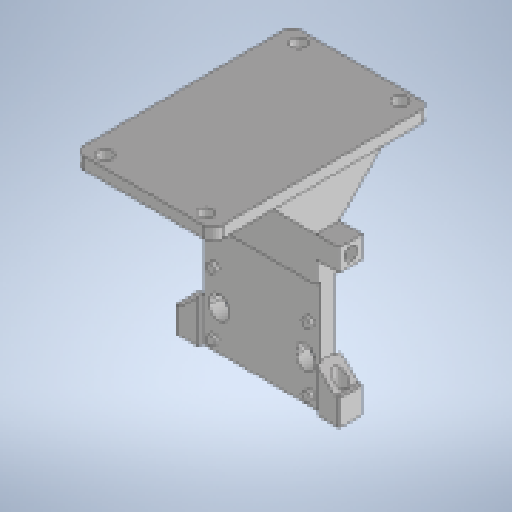
# Autodesk Inventor part: cameraholder
Saved by Autodesk Inventor 2025.1 (Build 291241000, 241)
## iProperties
Created: 2026-04-04
Part Number: cameraholder
Material: Generic
Document SubType Name: Modeling
Designer: User
Density: 1 g/cm^3
Appearance: Default
Author: User
## iProperties of the stored document cameraholder_3DPrint.ipt
Created: 2026-04-04
Part Number: cameraholder_3DPrint
Material: Generic
Document SubType Name: Modeling
Designer: User
Density: 1 g/cm^3
Appearance: Default
Author: User
Autodesk Inventor part; units mm, degrees
ref_plane "YZ Plane" through (0, 0, 0) normal (1, 0, 0) x (0, 1, 0)
sketch "Sketch1" plane through (0, 0, 0) normal (0, 0, 1) x (1, 0, 0)
  circle A0 centre (10.25, -9.75) radius 1.1 projected
  circle A1 centre (-10.25, -9.75) radius 1.1 projected
  circle A2 centre (-10.25, 3.75) radius 1.1 projected
  circle A3 centre (10.25, 3.75) radius 1.1 projected
  circle A4 centre (9.25, -4) radius 1.5 projected
  circle A5 centre (-9.25, -4) radius 1.5 projected
  arc A6 (7.25, -4) -> (11.25, -4) centre (9.25, -4) ccw
  arc A7 (-11.25, -4) -> (-7.25, -4) centre (-9.25, -4) ccw
  line L0 (8.2, -12) -> (-8.2, -12) projected
  line L1 (12.5, 1) -> (12.5, -7.7) projected
  line L2 (-12.5, 12) -> (12.5, 12) projected
  line L3 (-12.5, -7.7) -> (-12.5, 1) projected
  line L4 (12.5, -12) -> (-12.5, -12)
  line L5 (-12.5, -12) -> (-12.5, 12)
  line L6 (-12.5, 12) -> (12.5, 12)
  line L7 (12.5, 12) -> (12.5, -12)
  line L8 (-9.25, -4) -> (-9.25, -3)
  line L9 (9.25, -4) -> (9.25, -3)
  line L10 (-11.25, -4) -> (-11.25, -3)
  line L11 (-7.25, -4) -> (-7.25, -3)
  line L12 (7.25, -4) -> (7.25, -3)
  line L13 (11.25, -4) -> (11.25, -3)
  arc A8 (-9.25, -5) -> (-7.7976, -4.375) centre (-9.25, -3) ccw
  arc A9 (-7.25, -3) -> (-11.25, -3) centre (-9.25, -3) ccw
  arc A10 (9.25, -5) -> (10.7024, -4.375) centre (9.25, -3) ccw
  arc A11 (11.25, -3) -> (7.25, -3) centre (9.25, -3) ccw
  point P0 (0, 0)
  dimension "d0" = 0.5
  dimension "d1" = 0.5
  dimension "d70" = 1
  dimension "d74" = 3.25
  constraints: 20 end point, 12 point on circle, 6 centre point, 6 tangent, 4 vertical, 3 parallel, 2 point on line, 1 horizontal, 1 perpendicular, 4 other
  measures "d70" distance of L8.start L8.end
  measures "d74" distance from line of L1 L9.end
extrude "Extrusion1" add sketch "Sketch1" along normal blind 3 contours L0 L4 L5 L3 L2 L7 L1
sketch "Sketch2" plane through (-12.5, 12, 0) normal (0, 1, 0) x (1, 0, 0)
  line L0 (25, 0) -> (0, 0) projected
  line L1 (0, 0) -> (0, -3) projected
  line L2 (25, -3) -> (0, -3) projected
  line L3 (25, 0) -> (25, -3) projected
  point P0 (12.5, 0)
extrude "Extrusion2" add sketch "Sketch2" along normal blind 2
sketch "Sketch3" plane through (-12.5, 14, 0) normal (0, 1, 0) x (1, 0, 0)
  line L0 (0, 1) -> (25, 1) projected
  line L1 (25, 0) -> (0, 0) projected
  line L2 (0, -3) -> (25, -3) projected
  line L3 (0, -4) -> (25, -4)
  line L4 (0, 1) -> (25, 1)
  line L5 (25, 1) -> (25, -4)
  line L6 (25, -4) -> (0, -4)
  line L7 (0, -4) -> (0, 1)
  point P0 (12.5, 0)
  dimension "d6" = 1
  constraints: 10 end point, 3 parallel, 1 horizontal, 1 perpendicular
  measures "d6" distance between parallel lines of L2 L3
extrude "Extrusion3" add sketch "Sketch3" along normal blind 7.5
sketch "Sketch8" plane through (-12.5, -12, 0) normal (-1, 0, 0) x (0, 0, 1)
  line L0 (4, 24) -> (3, 24)
  line L1 (3, 26) -> (4, 26) projected
  line L2 (3, 0) -> (3, 26) projected
  line L3 (0, 0) -> (0, 26) projected
  line L4 (-1, 26) -> (0, 26) projected
  line L5 (4, 24.1) -> (3, 24.1)
  line L6 (4, 24.1) -> (-1, 24.1)
  line L7 (0, 24.1) -> (-1, 24.1)
  line L8 (-1, 24.1) -> (-1, 26)
  line L9 (-1, 26) -> (0, 26)
  line L10 (0, 26) -> (0, 24.1)
  line L11 (3, 24.1) -> (4, 24.1)
  line L12 (4, 24.1) -> (4, 26)
  line L13 (4, 26) -> (3, 26)
  line L14 (3, 26) -> (3, 24.1)
  point P0 (0, 12)
  dimension "d22" = 0.1
  constraints: 22 end point, 5 parallel, 4 horizontal, 2 perpendicular, 2 point on line, 2 other
  measures "d22" distance between parallel lines of L0 L5
extrude "Extrusion7" add sketch "Sketch8" against normal up to surface (25 mm away)
sketch "Sketch9" plane through (0, 0, 3) normal (0, 0, 1) x (1, 0, 0)
  circle A0 centre (10.25, -9.75) radius 1.1
  circle A1 centre (10.25, 3.75) radius 1.1
  circle A2 centre (-10.25, 3.75) radius 1.1
  circle A3 centre (-10.25, -9.75) radius 1.1
  circle A4 centre (-10.25, -9.75) radius 1
  circle A5 centre (-10.25, 3.75) radius 1
  circle A6 centre (10.25, 3.75) radius 1
  circle A7 centre (10.25, -9.75) radius 1
  point P0 (0, 0)
  dimension "d25" = 0.1
  dimension "d26" = 0.1
  dimension "d27" = 0.1
  dimension "d28" = 0.1
  constraints: 8 centre point, 8 other
  measures "d25" radial gap between concentric circles of A3 A4
  measures "d26" radial gap between concentric circles of A2 A5
  measures "d27" radial gap between concentric circles of A1 A6
  measures "d28" radial gap between concentric circles of A0 A7
ref_plane "Work Plane1" through (-12.5, 0.8429, -0.9) normal (0, 0, -1) x (0, 1, 0)
extrude "Extrusion8" add sketch "Sketch9" against normal up to surface (3.9 mm away) contours A4 | A5 | A6 | A7
sketch "Sketch10" plane through (-10.25, 3.75, 3) normal (0, 0, 1) x (1, 0, 0)
  circle A0 centre (0, 0) radius 1.1
  circle A1 centre (0, -13.5) radius 1.1
  circle A2 centre (20.5, -13.5) radius 1.1
  circle A3 centre (20.5, 0) radius 1.1
  point P0 (10.25, -3.75)
  constraints: 4 centre point, 8 other
extrude "Extrusion9" add sketch "Sketch10" against normal up to surface (3 mm away)
sketch "Sketch11" plane through (0, 0, 3) normal (0, 0, 1) x (1, 0, 0)
  circle A0 centre (10.25, -9.75) radius 1 projected
  circle A1 centre (10.25, 3.75) radius 1 projected
  circle A2 centre (-10.25, 3.75) radius 1 projected
  circle A3 centre (-10.25, -9.75) radius 1 projected
  point P0 (0, 0)
ref_plane "Work Plane2" through (8.65, 0.8429, 3.9) normal (0, 0, 1) x (1, 0, 0)
extrude "Extrusion10" add sketch "Sketch11" along normal up to surface (0.9 mm away)
sketch "Sketch12" plane through (-12.5, 21.5, 4) normal (0, 0, 1) x (1, 0, 0)
  line L0 (25, -9.4) -> (25, 0) projected
  line L1 (25, 0) -> (25, -4.7)
  line L2 (25, -4.7) -> (30, -4.7)
  line L3 (30, -4.7) -> (30, 0)
  line L4 (30, 0) -> (25, 0)
  line L5 (25, 0) -> (25, -4.7)
  line L6 (0, -9.4) -> (0, 0) projected
  line L7 (0, 0) -> (25, 0) projected
  line L8 (0, 0) -> (-5, 0)
  line L9 (-5, 0) -> (-5, -4.7)
  line L10 (-5, -4.7) -> (0, -4.7)
  line L11 (0, -4.7) -> (0, 0)
  point P0 (12.5, -21.5)
  dimension "d35" = 5
  dimension "d36" = 5
  constraints: 18 end point, 4 parallel, 2 horizontal, 2 perpendicular, 1 midpoint
  measures "d35" distance of L4.end L3.end
  measures "d36" distance of L10.end L9.end
extrude "Extrusion11" add sketch "Sketch12" against normal up to surface (5 mm away)
sketch "Sketch13" plane through (-12.5, -12, 0) normal (0, -1, 0) x (1, 0, 0)
  line L0 (0, 0) -> (0, 3) projected
  line L1 (25, 0) -> (25, 3) projected
  line L2 (25.2, 0) -> (25.2, 3)
  line L3 (-0.2, 0) -> (-0.2, 3)
  line L4 (-5, 4) -> (-5, -1) projected
  line L5 (-5, -1) -> (0, -1) projected
  line L6 (-5, 4) -> (0, 4) projected
  line L7 (25, -1) -> (30, -1) projected
  line L8 (30, 4) -> (30, -1) projected
  line L9 (25, 4) -> (30, 4) projected
  line L10 (30, -1) -> (25.2, -1)
  line L11 (25.2, -1) -> (25.2, 4)
  line L12 (25.2, 4) -> (30, 4)
  line L13 (30, 4) -> (30, -1)
  line L14 (-5, -1) -> (-0.2, -1)
  line L15 (-0.2, -1) -> (-0.2, 4)
  line L16 (-0.2, 4) -> (-5, 4)
  line L17 (-5, 4) -> (-5, -1)
  line L18 (0, 0) -> (25, 0) projected
  line L19 (0, 0) -> (-0.2, 0)
  line L20 (0, 3) -> (-0.2, 3)
  line L21 (25, -1) -> (25, 0) projected
  line L22 (25, 0) -> (25.2, 0)
  line L23 (25, 3) -> (25.2, 3)
  point P0 (12.5, 0)
  point P1 (-0.2, 3)
  point P2 (-0.2, 0)
  dimension "d39" = 0.2
  dimension "d40" = 0.2
  constraints: 28 end point, 7 parallel, 4 perpendicular, 2 horizontal, 2 point on line, 1 collinear
  measures "d39" distance between parallel lines of L1 L2
  measures "d40" distance between parallel lines of L0 L3
extrude "Extrusion12" add sketch "Sketch13" against normal blind 5.5 contours L19 L3 L20 L0 | L15 L5 L4 L6 L3 | L1 L23 L2 L22 | L2 L11 L9 L8 L7
sketch "Sketch14" plane through (-12.5, -6.5, 0) normal (0, 1, 0) x (1, 0, 0)
  circle A0 centre (-2.6, -1.5) radius 1.5
  circle A1 centre (27.6, -1.5) radius 1.5
  circle A2 centre (27.6, -1.5) radius 1.4
  circle A3 centre (-2.6, -1.5) radius 1.4
  point P0 (12.5, 0)
  dimension "d43" = 0.1
  dimension "d44" = 0.1
  constraints: 4 centre point, 4 other
  measures "d43" radial gap between concentric circles of A1 A2
  measures "d44" radial gap between concentric circles of A0 A3
extrude "Extrusion13" cut sketch "Sketch14" against normal blind 5.5 contours A2 | A3
chamfer "Chamfer3" distance 0.2 angle 45 8 edges at (-12.7, -9.25, 4) (-17.5, -9.25, 4) (-12.7, -9.25, -1) (-17.5, -9.25, -1) (17.5, -9.25, 4) (12.7, -9.25, 4) (17.5, -9.25, -1) (12.7, -9.25, -1)
chamfer "Chamfer4" distance 3.9999 angle 45 2 edges at (-12.5, -6.5, 1.5) (12.5, -6.5, 1.5)
sketch "Sketch15" plane through (-17.5, 16.8, 4) normal (-1, 0, 0) x (0, 0, 1)
  circle A0 centre (-2.5, 2.35) radius 1.5
  circle A1 centre (-2.5, 2.35) radius 1.4
  point P0 (-4, -16.8)
  dimension "d53" = 0.1
  constraints: 2 centre point, 2 other
  measures "d53" radial gap between concentric circles of A0 A1
extrude "Extrusion14" cut sketch "Sketch15" against normal blind 5.5 contours A1
sketch "Sketch16" plane through (17.5, 16.8, 4) normal (1, 0, 0) x (0, 0, -1)
  circle A0 centre (2.5, 2.35) radius 1.4 projected
  point P0 (4, -16.8)
extrude "Extrusion15" cut sketch "Sketch16" against normal blind 5.5
sketch "Sketch17" plane through (-12.5, 12.1, 4) normal (0, 0, 1) x (1, 0, 0)
  line L0 (25, 0) -> (25, 4.7) projected
  line L1 (0, 0) -> (0, 4.7) projected
  line L2 (30, 9.4) -> (-5, 9.4) projected
  line L3 (24.5905, 22.6402) -> (-1.0328, 22.6402)
  line L4 (25, 9.4) -> (0, 9.4)
  line L5 (0, 9.4) -> (0, 22.6402)
  line L6 (0, 22.6402) -> (25, 22.6402)
  line L7 (25, 22.6402) -> (25, 9.4)
  point P0 (12.5, -12.1)
  dimension "d58" = 25
  constraints: 10 end point, 2 horizontal, 2 parallel, 2 point on line, 1 perpendicular, 2 other
  measures "d58" distance of L5.end L6.end
extrude "Extrusion16" add sketch "Sketch17" against normal up to surface (5 mm away)
sketch "Sketch18" plane through (-12.5, 34.7402, 4) normal (0, 1, 0) x (1, 0, 0)
  circle A0 centre (22.5429, 20.4577) radius 1.5 construction
  circle A1 centre (22.5429, 20.4577) radius 1.5
  circle A2 centre (0.9195, 20.4343) radius 1.5
  circle A3 centre (22.5878, -21.1423) radius 1.5
  circle A4 centre (0.9645, -21.1657) radius 1.5
  line L0 (24.5905, -23.6401) -> (-1.0328, -23.6678)
  arc A5 (24.5905, -23.6401) -> (26.5884, -21.638) centre (24.5884, -21.6401) ccw
  line L1 (26.5873, -20.638) -> (26.5884, -21.638)
  arc A6 (-3.035, -21.67) -> (-1.0328, -23.6678) centre (-1.035, -21.6678) ccw
  line L2 (-3.035, -21.67) -> (-3.0361, -20.67)
  line L3 (26.5423, 20.962) -> (26.5434, 19.962)
  arc A7 (26.5423, 20.962) -> (24.5402, 22.9598) centre (24.5423, 20.9598) ccw
  line L4 (-1.0832, 22.9321) -> (24.5402, 22.9598)
  line L5 (-1.0832, 22.9321) -> (24.5402, 22.9598)
  arc A8 (-1.0832, 22.9321) -> (-3.081, 20.93) centre (-1.081, 20.9321) ccw
  line L6 (-3.08, 19.93) -> (-3.081, 20.93)
  line L7 (-3.08, 19.93) -> (-3.0361, -20.67)
  line L8 (26.5434, 19.962) -> (26.5873, -20.638)
  point P0 (12.5, 4)
  constraints: 18 end point, 9 centre point, 8 point on circle, 2 collinear, 37 other
extrude "Extrusion17" add sketch "Sketch18" against normal blind 2.5
sketch "Sketch19" plane through (12.5, 21.5, 4) normal (1, 0, 0) x (0, 0, -1)
  line L0 (5, 0) -> (5, 10.7402) projected
  line L1 (0, 0) -> (0, 10.7402) projected
  line L2 (20.962, 10.7402) -> (-21.638, 10.7402) projected
  line L3 (0, 10.7402) -> (5, 10.7402) projected
  circle A0 centre (5, 10.7402) radius 10.7402
  circle A1 centre (0, 10.7402) radius 10.7402
  line L4 (5, 0) -> (15.7402, 10.7402)
  line L5 (0, 0) -> (-10.7402, 10.7402)
  point P0 (4, -21.5)
  constraints: 4 end point, 4 point on circle, 2 centre point, 2 coincident, 2 point on line
extrude "Extrusion18" add sketch "Sketch19" against normal blind 2.5 contours L0 A1 L2 L4 | L0 L2 A1 | A0 L2 L1 | L1 L5 L2 A0
sketch "Sketch20" plane through (-12.5, 21.5, -1) normal (-1, 0, 0) x (0, 0, 1)
  line L0 (5, 10.7402) -> (15.7402, 10.7402) projected
  line L1 (5, 0) -> (5, 10.7402) projected
  line L2 (5, 0) -> (15.7402, 10.7402) projected
  line L3 (-10.7402, 10.7402) -> (0, 10.7402) projected
  line L4 (-10.7402, 10.7402) -> (0, 0) projected
  line L5 (0, 10.7402) -> (0, 0) projected
  point P0 (1, -21.5)
extrude "Extrusion19" add sketch "Sketch20" against normal blind 2.5
chamfer "Chamfer5" distance 2 angle 45 6 edges at (0, 32.2402, -1) (0, 32.2402, 4) (-10, 32.2402, -6.3701) (10, 32.2402, -6.3701) (-10, 32.2402, 9.3701) (10, 32.2402, 9.3701)
sketch "Sketch21" plane through (-12.5, 32.2402, 4) normal (0, -1, 0) x (1, 0, 0)
  line L0 (20.5, -7) -> (20.5, -15.7402) projected
  line L1 (20.5, -7) -> (4.5, -7)
  line L2 (4.5, -15.7402) -> (4.5, -7) projected
  line L3 (-1.0832, -22.9321) -> (24.5402, -22.9598) projected
  line L4 (15.5, -15.7402) -> (15.5, -12)
  line L5 (14.0037, -12) -> (11, -12)
  line L6 (-1.0778, -17.9321) -> (24.5456, -17.9598)
  line L7 (14.0037, -12) -> (11, -12)
  line L8 (9.5, -17.9436) -> (15.5, -17.9436)
  line L9 (15.5, -15.7402) -> (15.5, -12)
  line L10 (-1.0751, -15.4321) -> (24.5483, -15.4598)
  line L11 (12.5, -17.9436) -> (15.5, -15.4501)
  line L12 (12.5, -17.9436) -> (9.5, -15.4436)
  line L13 (14, -15.4484) -> (14.0037, -12)
  line L14 (11, -15.4452) -> (11, -12)
  line L15 (15.5, -15.4501) -> (14, -15.4484)
  line L16 (9.5, -15.4436) -> (11, -15.4452)
  line L17 (14, -15.4484) -> (15.5, -15.4501)
  point P0 (12.5, -4)
  dimension "d75" = 5
  dimension "d76" = 5
  dimension "d79" = 2.5
  constraints: 30 end point, 6 point on line, 3 parallel, 2 collinear, 2 horizontal, 1 midpoint, 1 perpendicular, 2 other
  measures "d75" distance between parallel lines of L0 L4
  measures "d76" distance between parallel lines of L3 L6
  measures "d79" distance between parallel lines of L6 L10
extrude "Extrusion20" cut sketch "Sketch21" against normal blind 0.5 contours L11 L12 L10 | L10 L14 L5 L13
body "Solid1"
